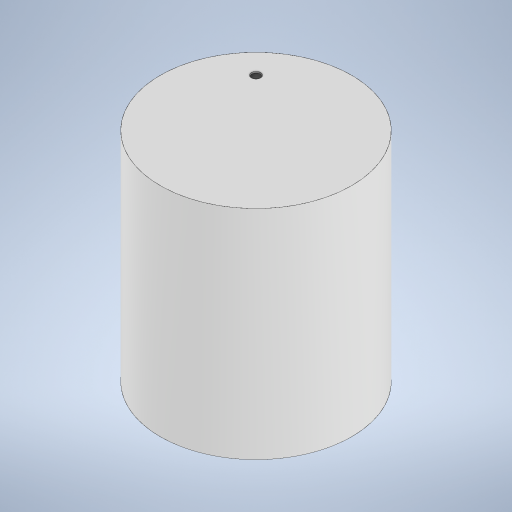
# Autodesk Inventor part: FermentingTun
Saved by Autodesk Inventor 2024 (Build 280153000, 153)
## iProperties
Created: 2025-09-20
Part Number: FermentingTun
Material: Generic
Document SubType Name: Modeling
Designer: Emil
Density: 1 g/cm^3
Appearance: Default
Author: Emil
Autodesk Inventor part; units mm, degrees
ref_plane "YZ Plane" through (0, 0, 0) normal (1, 0, 0) x (0, 1, 0)
ref_plane "XZ Plane" through (0, 0, 0) normal (0, 1, 0) x (-1, 0, 0)
ref_plane "XY Plane" through (0, 0, 0) normal (0, 0, 1) x (1, 0, 0)
sketch "Sketch1" plane through (0, 0, 0) normal (0, 1, 0) x (-1, 0, 0)
  circle A0 centre (0, 0) radius 142.5
  circle A1 centre (0, 0) radius 139
  dimension "d0" = 285
  dimension "d1" = 278
  constraints: 2 centre point, 2 coincident
  measures "d0" diameter of A0
  measures "d1" diameter of A1
extrude "Extrusion1" add sketch "Sketch1" along normal blind 320
sketch "Sketch2" plane through (0, 0, 0) normal (0, -1, 0) x (1, 0, 0)
  circle A0 centre (0, 0) radius 142.5
  constraints: 1 centre point, 1 coincident
extrude "Extrusion2" add sketch "Sketch2" along normal blind 2
sketch "Sketch3" plane through (0, 320, 0) normal (0, 1, 0) x (1, 0, 0)
  circle A0 centre (0, 0) radius 142.5
  constraints: 1 centre point, 1 coincident
extrude "Extrusion3" add sketch "Sketch3" along normal blind 2
sketch "Sketch4" plane through (0, 322, 0) normal (0, 1, 0) x (1, 0, 0)
  circle A0 centre (0, 0) radius 142.5 construction
  line L0 (0, -142.5) -> (0, 142.5) construction
  line L1 (-142.5, 0) -> (142.5, 0) construction
  line L2 (0, 142.5) -> (-142.5, 0) construction
  line L3 (0, 0) -> (-98.2878, 98.2878) construction
  circle A1 centre (0, 0) radius 139 construction
  circle A2 centre (-71.25, 71.25) radius 7
  dimension "d8" = 14
  constraints: 8 end point, 4 point on circle, 2 perpendicular, 1 centre point, 1 midpoint, 1 point on line, 1 vertical, 2 other
  measures "d8" diameter of A2
extrude "Extrusion9" cut sketch "Sketch4" against normal blind 10
body "Solid1"
